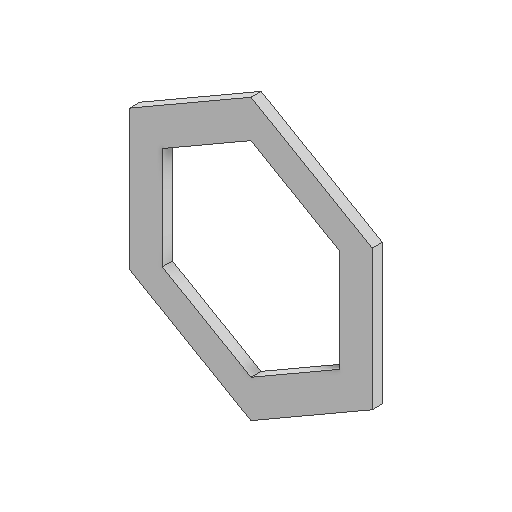
# Autodesk Inventor part: Shaft Spacers V2
Saved by Autodesk Inventor 2024.1 (Build 281209000, 209)
## iProperties
Created: 2023-10-24
Part Number: Shaft Spacers V2
Material: Generic
Document SubType Name: Modeling
Designer: david
Density: 1 g/cm^3
Appearance: Default
Author: david
Autodesk Inventor part; units mm, degrees
ref_plane "YZ Plane" through (0, 0, 0) normal (1, 0, 0) x (0, 1, 0)
ref_plane "XZ Plane" through (0, 0, 0) normal (0, 1, 0) x (-1, 0, 0)
ref_plane "XY Plane" through (0, 0, 0) normal (0, 0, 1) x (1, 0, 0)
sketch "Sketch1" plane through (0, 0, 0) normal (0, 0, 1) x (1, 0, 0)
  line L0 (0, 7.5633) -> (6.55, 3.7816)
  line L1 (6.55, 3.7816) -> (6.55, -3.7816)
  line L2 (6.55, -3.7816) -> (0, -7.5633)
  line L3 (0, -7.5633) -> (-6.55, -3.7816)
  line L4 (-6.55, -3.7816) -> (-6.55, 3.7816)
  line L5 (-6.55, 3.7816) -> (0, 7.5633)
  line L6 (-8.95, 5.1673) -> (-8.95, -5.1673)
  line L7 (-8.95, -5.1673) -> (0, -10.3346)
  line L8 (0, -10.3346) -> (8.95, -5.1673)
  line L9 (8.95, -5.1673) -> (8.95, 5.1673)
  line L10 (8.95, 5.1673) -> (0, 10.3346)
  line L11 (0, 10.3346) -> (-8.95, 5.1673)
  point P0 (0, 0)
  point P1 (0, 0)
  point P2 (-6.55, 0)
  dimension "d0" = 13.1
  dimension "d1" = 2.4
  constraints: 24 end point, 1 coincident, 1 midpoint, 18 other
  measures "d0" distance between parallel lines of L1 L4
  measures "d1" distance from line of L6 point (-6.55, 0)
extrude "Extrusion1" add sketch "Sketch1" along normal blind 0.75
body "Solid1"
